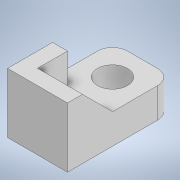
# Autodesk Inventor part: 零件2
Saved by Autodesk Inventor 2020 (Build 240168000, 168)
## iProperties
Created: 2020-09-19
Part Number: 零件2
Material: 一般
Document SubType Name: Modeling
Designer: User
Density: 1 g/cm^3
Appearance: 預設
Author: User
Autodesk Inventor part; units mm, degrees
ref_plane "YZ Plane" through (0, 0, 0) normal (1, 0, 0) x (0, 1, 0)
ref_plane "XZ Plane" through (0, 0, 0) normal (0, 1, 0) x (-1, 0, 0)
ref_plane "XY Plane" through (0, 0, 0) normal (0, 0, 1) x (1, 0, 0)
sketch "草圖1" plane through (0, 0, 0) normal (0, 1, 0) x (-1, 0, 0)
  line L0 (0, 0) -> (40, 0)
  line L1 (40, 0) -> (40, -60)
  line L2 (30, -70) -> (10, -70)
  line L3 (0, -60) -> (0, 0)
  circle A0 centre (20, -50) radius 10
  arc A1 (30, -70) -> (40, -60) centre (30, -60) ccw
  arc A2 (0, -60) -> (10, -70) centre (10, -60) ccw
  line L4 (0, -10) -> (30, -10)
  line L5 (30, -10) -> (30, -30)
  line L6 (30, -30) -> (40, -30)
  point P0 (40, -70)
  point P1 (0, -70)
  point P2 (40, -10)
  point P3 (0, -30)
  dimension "d0" = 40
  dimension "d1" = 70
  dimension "d5" = 20
  dimension "d6" = 20
  dimension "d7" = 20
  dimension "d8" = 10
  dimension "d18" = 30
  dimension "d19" = 20
  dimension "d20" = 10
  constraints: 14 end point, 6 point on line, 4 point on circle, 4 tangent, 3 centre point, 2 horizontal, 2 midpoint, 2 parallel, 2 perpendicular, 1 equal radius, 1 vertical
  measures "d0" distance of point (40, -70) point (0, -70)
  measures "d1" distance of L0.end point (40, -70)
  measures "d5" diameter of A0
  measures "d6" distance from line of L2 A0.centre
  measures "d7" distance from line of L1 A0.centre
  measures "d8" radius of A1
  measures "d18" distance of L4.start L4.end
  measures "d19" distance of L4.end L5.end
  measures "d20" distance between parallel lines of L4 L0
extrude "擠出1" add sketch "草圖1" along normal blind 40 contours L0 L1 L6 L5 L4 L3
extrude "擠出2" add sketch "草圖1" along normal blind 20
sketch "草圖3" plane through (0, 0, 0) normal (1, 0, 0) x (0, 0, -1)
  line L0 (10, 40) -> (30, 20)
  line L1 (10, 20) -> (10, 40) projected
  line L2 (30, 20) -> (10, 20)
  line L3 (10, 20) -> (10, 40)
  point P0 (0, 0)
  constraints: 6 end point, 1 collinear, 1 perpendicular
extrude "擠出4" add sketch "草圖3" against normal blind 10
